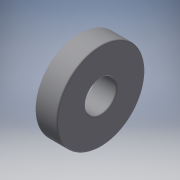
# Autodesk Inventor part: rbearing2
Saved by Autodesk Inventor 2019 (Build 230136000, 136)
## iProperties
Shininess: 64.0
Angle Display Precision: 2
Document Length Units: 11269
Document Angle Units: 11279
Document Time Units: 11290
Document Mass Units: 11283
Document Length Units Precision: 3
Document Angle Units Precision: 2
Compacted: True
Created: 2005-03-18
Part Number: rbearing2
Document SubType Name: Modeling
Designer: Miroslav Petele
Density: 1 g/cm^3
Material: Generic
Appearance: Default
Density: 0.0
Volumn: 0.0
Area: 0.0
PropertySet Name: Model Information
Control State: 0
Master: False
Checked Out: False
Author: Miroslav Petele
Autodesk Inventor part; units mm, degrees
ref_plane "YZ Plane" through (0, 0, 0) normal (1, 0, 0) x (0, 1, 0)
ref_plane "XZ Plane" through (0, 0, 0) normal (0, 1, 0) x (-1, 0, 0)
ref_plane "XY Plane" through (0, 0, 0) normal (0, 0, 1) x (1, 0, 0)
sketch "Sketch1" plane through (0, 0, 0) normal (0, 0, 1) x (1, 0, 0)
  line L0 (-4.4603, 0) -> (31.4603, 0) projected
  line L1 (0, 10.5397) -> (0, 56.9603) projected
  spline S0 degree 2 poles (2.5, 17.5) (1.1287, 17.6287) (1, 19) knots 0 0 0 1 1 1
  spline S1 degree 2 poles (1, 19) (1, 33.75) (1, 48.5) knots 0 0 0 1 1 1
  spline S2 degree 2 poles (1, 48.5) (1.1287, 49.8713) (2.5, 50) knots 0 0 0 1 1 1
  spline S3 degree 2 poles (2.5, 50) (13.5, 50) (24.5, 50) knots 0 0 0 1 1 1
  spline S4 degree 2 poles (24.5, 50) (25.8713, 49.8713) (26, 48.5) knots 0 0 0 1 1 1
  spline S5 degree 2 poles (26, 48.5) (26, 33.75) (26, 19) knots 0 0 0 1 1 1
  spline S6 degree 2 poles (26, 19) (25.8713, 17.6287) (24.5, 17.5) knots 0 0 0 1 1 1
  spline S7 degree 2 poles (24.5, 17.5) (23.8529, 17.5) (23.2059, 17.5) knots 0 0 0 1 1 1
  spline S8 degree 2 poles (23.2059, 17.5) (22.5588, 17.5) (21.9118, 17.5) knots 0 0 0 1 1 1
  spline S9 degree 2 poles (21.9118, 17.5) (21.2647, 17.5) (20.6176, 17.5) knots 0 0 0 1 1 1
  spline S10 degree 2 poles (20.6176, 17.5) (19.9706, 17.5) (19.3235, 17.5) knots 0 0 0 1 1 1
  spline S11 degree 2 poles (19.3235, 17.5) (18.6765, 17.5) (18.0294, 17.5) knots 0 0 0 1 1 1
  spline S12 degree 2 poles (18.0294, 17.5) (17.3824, 17.5) (16.7353, 17.5) knots 0 0 0 1 1 1
  spline S13 degree 2 poles (16.7353, 17.5) (16.0882, 17.5) (15.4412, 17.5) knots 0 0 0 1 1 1
  spline S14 degree 2 poles (15.4412, 17.5) (14.7941, 17.5) (14.1471, 17.5) knots 0 0 0 1 1 1
  spline S15 degree 2 poles (14.1471, 17.5) (13.5, 17.5) (12.8529, 17.5) knots 0 0 0 1 1 1
  spline S16 degree 2 poles (12.8529, 17.5) (12.2059, 17.5) (11.5588, 17.5) knots 0 0 0 1 1 1
  spline S17 degree 2 poles (11.5588, 17.5) (10.9118, 17.5) (10.2647, 17.5) knots 0 0 0 1 1 1
  spline S18 degree 2 poles (10.2647, 17.5) (9.6176, 17.5) (8.9706, 17.5) knots 0 0 0 1 1 1
  spline S19 degree 2 poles (8.9706, 17.5) (8.3235, 17.5) (7.6765, 17.5) knots 0 0 0 1 1 1
  spline S20 degree 2 poles (7.6765, 17.5) (7.0294, 17.5) (6.3824, 17.5) knots 0 0 0 1 1 1
  spline S21 degree 2 poles (6.3824, 17.5) (5.7353, 17.5) (5.0882, 17.5) knots 0 0 0 1 1 1
  spline S22 degree 2 poles (5.0882, 17.5) (4.4412, 17.5) (3.7941, 17.5) knots 0 0 0 1 1 1
  spline S23 degree 2 poles (3.7941, 17.5) (3.1471, 17.5) (2.5, 17.5) knots 0 0 0 1 1 1
  point P0 (1.4393, 17.9393)
  point P1 (1, 33.75)
  point P2 (1.4393, 49.5607)
  point P3 (13.5, 50)
  point P4 (25.5607, 49.5607)
  point P5 (26, 33.75)
  point P6 (25.5607, 17.9393)
  point P7 (23.8529, 17.5)
  point P8 (22.5588, 17.5)
  point P9 (21.2647, 17.5)
  point P10 (19.9706, 17.5)
  point P11 (18.6765, 17.5)
  point P12 (17.3824, 17.5)
  point P13 (16.0882, 17.5)
  point P14 (14.7941, 17.5)
  point P15 (13.5, 17.5)
  point P16 (12.2059, 17.5)
  point P17 (10.9118, 17.5)
  point P18 (9.6176, 17.5)
  point P19 (8.3235, 17.5)
  point P20 (7.0294, 17.5)
  point P21 (5.7353, 17.5)
  point P22 (4.4412, 17.5)
  point P23 (3.1471, 17.5)
  dimension "d0" = 2.5
  dimension "d1" = 17.5
  dimension "d2" = 1.4393
  dimension "d3" = 17.9393
  dimension "d4" = 1
  dimension "d5" = 19
  dimension "d6" = 1
  dimension "d7" = 33.75
  dimension "d8" = 1
  dimension "d9" = 48.5
  dimension "d10" = 1.4393
  dimension "d11" = 49.5607
  dimension "d12" = 2.5
  dimension "d13" = 50
  dimension "d14" = 13.5
  dimension "d15" = 50
  dimension "d16" = 24.5
  dimension "d17" = 50
  dimension "d18" = 25.5607
  dimension "d19" = 49.5607
  dimension "d20" = 26
  dimension "d21" = 48.5
  dimension "d22" = 26
  dimension "d23" = 33.75
  dimension "d24" = 26
  dimension "d25" = 19
  dimension "d26" = 25.5607
  dimension "d27" = 17.9393
  dimension "d28" = 24.5
  dimension "d29" = 17.5
  dimension "d30" = 23.8529
  dimension "d31" = 17.5
  dimension "d32" = 23.2059
  dimension "d33" = 17.5
  dimension "d34" = 22.5588
  dimension "d35" = 17.5
  dimension "d36" = 21.9118
  dimension "d37" = 17.5
  dimension "d38" = 21.2647
  dimension "d39" = 17.5
  dimension "d40" = 20.6177
  dimension "d41" = 17.5
  dimension "d42" = 19.9706
  dimension "d43" = 17.5
  dimension "d44" = 19.3235
  dimension "d45" = 17.5
  dimension "d46" = 18.6765
  dimension "d47" = 17.5
  dimension "d48" = 18.0294
  dimension "d49" = 17.5
  dimension "d50" = 17.3823
  dimension "d51" = 17.5
  dimension "d52" = 16.7353
  dimension "d53" = 17.5
  dimension "d54" = 16.0882
  dimension "d55" = 17.5
  dimension "d56" = 15.4412
  dimension "d57" = 17.5
  dimension "d58" = 14.7941
  dimension "d59" = 17.5
  dimension "d60" = 14.1471
  dimension "d61" = 17.5
  dimension "d62" = 13.5
  dimension "d63" = 17.5
  constraints: 72 other
  measures "d0" distance from line of L1 point (2.5, 17.5)
  measures "d1" distance from line of L0 point (2.5, 17.5)
  measures "d2" distance from line of L1 point (1.439, 17.939)
  measures "d3" distance from line of L0 point (1.439, 17.939)
  measures "d4" distance from line of L1 point (1, 19)
  measures "d5" distance from line of L0 point (1, 19)
  measures "d6" distance from line of L1 point (1, 33.75)
  measures "d7" distance from line of L0 point (1, 33.75)
  measures "d8" distance from line of L1 point (1, 48.5)
  measures "d9" distance from line of L0 point (1, 48.5)
  measures "d10" distance from line of L1 point (1.439, 49.561)
  measures "d11" distance from line of L0 point (1.439, 49.561)
  measures "d12" distance from line of L1 point (2.5, 50)
  measures "d13" distance from line of L0 point (2.5, 50)
  measures "d14" distance from line of L1 point (13.5, 50)
  measures "d15" distance from line of L0 point (13.5, 50)
  measures "d16" distance from line of L1 point (24.5, 50)
  measures "d17" distance from line of L0 point (24.5, 50)
  measures "d18" distance from line of L1 point (25.561, 49.561)
  measures "d19" distance from line of L0 point (25.561, 49.561)
  measures "d20" distance from line of L1 point (26, 48.5)
  measures "d21" distance from line of L0 point (26, 48.5)
  measures "d22" distance from line of L1 point (26, 33.75)
  measures "d23" distance from line of L0 point (26, 33.75)
  measures "d24" distance from line of L1 point (26, 19)
  measures "d25" distance from line of L0 point (26, 19)
  measures "d26" distance from line of L1 point (25.561, 17.939)
  measures "d27" distance from line of L0 point (25.561, 17.939)
  measures "d28" distance from line of L1 point (24.5, 17.5)
  measures "d29" distance from line of L0 point (24.5, 17.5)
  measures "d30" distance from line of L1 point (23.853, 17.5)
  measures "d31" distance from line of L0 point (23.853, 17.5)
  measures "d32" distance from line of L1 point (23.206, 17.5)
  measures "d33" distance from line of L0 point (23.206, 17.5)
  measures "d34" distance from line of L1 point (22.559, 17.5)
  measures "d35" distance from line of L0 point (22.559, 17.5)
  measures "d36" distance from line of L1 point (21.912, 17.5)
  measures "d37" distance from line of L0 point (21.912, 17.5)
  measures "d38" distance from line of L1 point (21.265, 17.5)
  measures "d39" distance from line of L0 point (21.265, 17.5)
  measures "d40" distance from line of L1 point (20.618, 17.5)
  measures "d41" distance from line of L0 point (20.618, 17.5)
  measures "d42" distance from line of L1 point (19.971, 17.5)
  measures "d43" distance from line of L0 point (19.971, 17.5)
  measures "d44" distance from line of L1 point (19.324, 17.5)
  measures "d45" distance from line of L0 point (19.324, 17.5)
  measures "d46" distance from line of L1 point (18.676, 17.5)
  measures "d47" distance from line of L0 point (18.676, 17.5)
  measures "d48" distance from line of L1 point (18.029, 17.5)
  measures "d49" distance from line of L0 point (18.029, 17.5)
  measures "d50" distance from line of L1 point (17.382, 17.5)
  measures "d51" distance from line of L0 point (17.382, 17.5)
  measures "d52" distance from line of L1 point (16.735, 17.5)
  measures "d53" distance from line of L0 point (16.735, 17.5)
  measures "d54" distance from line of L1 point (16.088, 17.5)
  measures "d55" distance from line of L0 point (16.088, 17.5)
  measures "d56" distance from line of L1 point (15.441, 17.5)
  measures "d57" distance from line of L0 point (15.441, 17.5)
  measures "d58" distance from line of L1 point (14.794, 17.5)
  measures "d59" distance from line of L0 point (14.794, 17.5)
  measures "d60" distance from line of L1 point (14.147, 17.5)
  measures "d61" distance from line of L0 point (14.147, 17.5)
  measures "d62" distance from line of L1 point (13.5, 17.5)
  measures "d63" distance from line of L0 point (13.5, 17.5)
revolve "Revolution1" add sketch "Sketch1" angle 360 about axis through (-10, 0, 0) along (1, 0, 0)
equation "\"d0\" = MC_X1"
equation "\"d1\" = MC_Y1"
equation "\"d2\" = MC_X2"
equation "\"d3\" = MC_Y2"
equation "\"d4\" = MC_X3"
equation "\"d5\" = MC_Y3"
equation "\"d6\" = MC_X4"
equation "\"d7\" = MC_Y4"
equation "\"d8\" = MC_X5"
equation "\"d9\" = MC_Y5"
equation "\"d10\" = MC_X6"
equation "\"d11\" = MC_Y6"
equation "\"d12\" = MC_X7"
equation "\"d13\" = MC_Y7"
equation "\"d14\" = MC_X8"
equation "\"d15\" = MC_Y8"
equation "\"d16\" = MC_X9"
equation "\"d17\" = MC_Y9"
equation "\"d18\" = MC_X10"
equation "\"d19\" = MC_Y10"
equation "\"d20\" = MC_X11"
equation "\"d21\" = MC_Y11"
equation "\"d22\" = MC_X12"
equation "\"d23\" = MC_Y12"
equation "\"d24\" = MC_X13"
equation "\"d25\" = MC_Y13"
equation "\"d26\" = MC_X14"
equation "\"d27\" = MC_Y14"
equation "\"d28\" = MC_X15"
equation "\"d29\" = MC_Y15"
equation "\"d30\" = MC_X16"
equation "\"d31\" = MC_Y16"
equation "\"d32\" = MC_X17"
equation "\"d33\" = MC_Y17"
equation "\"d34\" = MC_X18"
equation "\"d35\" = MC_Y18"
equation "\"d36\" = MC_X19"
equation "\"d37\" = MC_Y19"
equation "\"d38\" = MC_X20"
equation "\"d39\" = MC_Y20"
equation "\"d40\" = MC_X21"
equation "\"d41\" = MC_Y21"
equation "\"d42\" = MC_X22"
equation "\"d43\" = MC_Y22"
equation "\"d44\" = MC_X23"
equation "\"d45\" = MC_Y23"
equation "\"d46\" = MC_X24"
equation "\"d47\" = MC_Y24"
equation "\"d48\" = MC_X25"
equation "\"d49\" = MC_Y25"
equation "\"d50\" = MC_X26"
equation "\"d51\" = MC_Y26"
equation "\"d52\" = MC_X27"
equation "\"d53\" = MC_Y27"
equation "\"d54\" = MC_X28"
equation "\"d55\" = MC_Y28"
equation "\"d56\" = MC_X29"
equation "\"d57\" = MC_Y29"
equation "\"d58\" = MC_X30"
equation "\"d59\" = MC_Y30"
equation "\"d60\" = MC_X31"
equation "\"d61\" = MC_Y31"
equation "\"d62\" = MC_X32"
equation "\"MC_X1\" = 2.5"
equation "\"MC_Y1\" = 17.5"
equation "\"MC_X2\" = 1.43934"
equation "\"MC_Y2\" = 17.93934"
equation "\"MC_X3\" = 1"
equation "\"MC_Y3\" = 19"
equation "\"MC_X4\" = 1"
equation "\"MC_Y4\" = 33.75"
equation "\"MC_X5\" = 1"
equation "\"MC_Y5\" = 48.5"
equation "\"MC_X6\" = 1.43934"
equation "\"MC_Y6\" = 49.56066"
equation "\"MC_X7\" = 2.5"
equation "\"MC_Y7\" = 50"
equation "\"MC_X8\" = 13.5"
equation "\"MC_Y8\" = 50"
equation "\"MC_X9\" = 24.5"
equation "\"MC_Y9\" = 50"
equation "\"MC_X10\" = 25.56066"
equation "\"MC_Y10\" = 49.56066"
equation "\"MC_X11\" = 26"
equation "\"MC_Y11\" = 48.5"
equation "\"MC_X12\" = 26"
equation "\"MC_Y12\" = 33.75"
equation "\"MC_X13\" = 26"
equation "\"MC_Y13\" = 19"
equation "\"MC_X14\" = 25.56066"
equation "\"MC_Y14\" = 17.93934"
equation "\"MC_X15\" = 24.5"
equation "\"MC_Y15\" = 17.5"
equation "\"MC_X16\" = 23.85294"
equation "\"MC_Y16\" = 17.5"
equation "\"MC_X17\" = 23.20588"
equation "\"MC_Y17\" = 17.5"
equation "\"MC_X18\" = 22.55882"
equation "\"MC_Y18\" = 17.5"
equation "\"MC_X19\" = 21.91176"
equation "\"MC_Y19\" = 17.5"
equation "\"MC_X20\" = 21.26471"
equation "\"MC_Y20\" = 17.5"
equation "\"MC_X21\" = 20.61765"
equation "\"MC_Y21\" = 17.5"
equation "\"MC_X22\" = 19.97059"
equation "\"MC_Y22\" = 17.5"
equation "\"MC_X23\" = 19.32353"
equation "\"MC_Y23\" = 17.5"
equation "\"MC_X24\" = 18.67647"
equation "\"MC_Y24\" = 17.5"
equation "\"MC_X25\" = 18.02941"
equation "\"MC_Y25\" = 17.5"
equation "\"MC_X26\" = 17.38235"
equation "\"MC_Y26\" = 17.5"
equation "\"MC_X27\" = 16.73529"
equation "\"MC_Y27\" = 17.5"
equation "\"MC_X28\" = 16.08824"
equation "\"MC_Y28\" = 17.5"
equation "\"MC_X29\" = 15.44118"
equation "\"MC_Y29\" = 17.5"
equation "\"MC_X30\" = 14.79412"
equation "\"MC_Y30\" = 17.5"
equation "\"MC_X31\" = 14.14706"
equation "\"MC_Y31\" = 17.5"
equation "\"MC_X32\" = 13.5"
equation "\"MC_Y32\" = 17.5"
equation "\"MC_X33\" = 12.85294"
equation "\"MC_Y33\" = 17.5"
equation "\"MC_X34\" = 12.20588"
equation "\"MC_Y34\" = 17.5"
equation "\"MC_X35\" = 11.55882"
equation "\"MC_Y35\" = 17.5"
equation "\"MC_X36\" = 10.91176"
equation "\"MC_Y36\" = 17.5"
equation "\"MC_X37\" = 10.26471"
equation "\"MC_Y37\" = 17.5"
equation "\"MC_X38\" = 9.61765"
equation "\"MC_Y38\" = 17.5"
equation "\"MC_X39\" = 8.97059"
equation "\"MC_Y39\" = 17.5"
equation "\"MC_X40\" = 8.32353"
equation "\"MC_Y40\" = 17.5"
equation "\"MC_X41\" = 7.67647"
equation "\"MC_Y41\" = 17.5"
equation "\"MC_X42\" = 7.02941"
equation "\"MC_Y42\" = 17.5"
equation "\"MC_X43\" = 6.38235"
equation "\"MC_Y43\" = 17.5"
equation "\"MC_X44\" = 5.73529"
equation "\"MC_Y44\" = 17.5"
equation "\"MC_X45\" = 5.08824"
equation "\"MC_Y45\" = 17.5"
equation "\"MC_X46\" = 4.44118"
equation "\"MC_Y46\" = 17.5"
equation "\"MC_X47\" = 3.79412"
equation "\"MC_Y47\" = 17.5"
equation "\"MC_X48\" = 3.14706"
equation "\"MC_Y48\" = 17.5"
body "Solid1"
